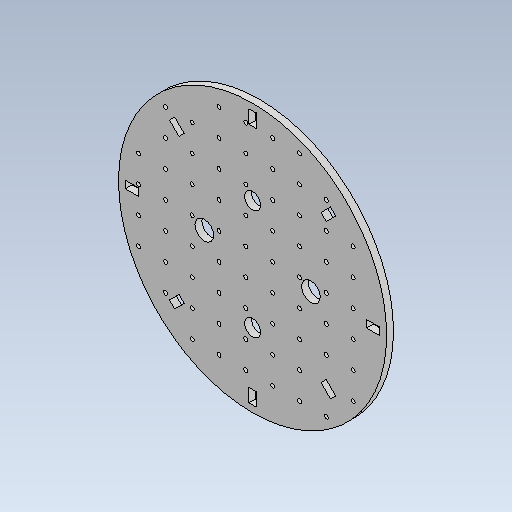
# Autodesk Inventor part: midPlate
Saved by Autodesk Inventor 2025 (Build 290162000, 162)
## iProperties
Created: 2024-08-12
Part Number: midPlate
Material: Polycarbonate, Clear
Document SubType Name: Modeling
Designer: PC
Density: 1.2 g/cm^3
Appearance: Default
Author: PC
Autodesk Inventor part; units mm, degrees
ref_plane "YZ Plane" through (0, 0, 0) normal (1, 0, 0) x (0, 1, 0)
ref_plane "XZ Plane" through (0, 0, 0) normal (0, 1, 0) x (-1, 0, 0)
ref_plane "XY Plane" through (0, 0, 0) normal (0, 0, 1) x (1, 0, 0)
sketch "Sketch1" plane through (0, 0, 0) normal (0, 0, 1) x (1, 0, 0)
  circle A0 centre (0, -18.52) radius 100
  line L0 (65, -83.52) -> (-65, -83.52) construction
  line L1 (-65, -83.52) -> (-65, 46.48) construction
  line L2 (-65, 46.48) -> (65, 46.48) construction
  line L3 (65, 46.48) -> (65, -83.52) construction
  line L4 (65, -83.52) -> (-65, 46.48) construction
  line L5 (-65, -83.52) -> (65, 46.48) construction
  line L6 (45, 26.48) -> (-45, 26.48) construction
  line L7 (-45, 26.48) -> (-45, -63.52) construction
  line L8 (-45, -63.52) -> (45, -63.52) construction
  line L9 (45, -63.52) -> (45, 26.48) construction
  line L10 (-25, 6.48) -> (25, 6.48) construction
  line L11 (25, 6.48) -> (25, -43.52) construction
  line L12 (25, -43.52) -> (-25, -43.52) construction
  line L13 (-25, -43.52) -> (-25, 6.48) construction
  line L14 (5, -13.52) -> (-5, -13.52) construction
  line L15 (-5, -13.52) -> (-5, -23.52) construction
  line L16 (-5, -23.52) -> (5, -23.52) construction
  line L17 (5, -23.52) -> (5, -13.52) construction
  circle A1 centre (-65, 46.48) radius 1.5
  circle A2 centre (-45, 46.48) radius 1.5
  circle A3 centre (-25, 46.48) radius 1.5
  circle A4 centre (-5, 46.48) radius 1.5
  circle A5 centre (15, 46.48) radius 1.5
  circle A6 centre (35, 46.48) radius 1.5
  circle A7 centre (55, 46.48) radius 1.5
  circle A8 centre (-65, 26.48) radius 1.5
  circle A9 centre (-65, 6.48) radius 1.5
  circle A10 centre (-65, -13.52) radius 1.5
  circle A11 centre (-65, -33.52) radius 1.5
  circle A12 centre (-65, -53.52) radius 1.5
  circle A13 centre (-65, -73.52) radius 1.5
  circle A14 centre (-45, 26.48) radius 1.5
  circle A15 centre (-25, 26.48) radius 1.5
  circle A16 centre (-5, 26.48) radius 1.5
  circle A17 centre (15, 26.48) radius 1.5
  circle A18 centre (35, 26.48) radius 1.5
  circle A19 centre (55, 26.48) radius 1.5
  circle A20 centre (-45, 6.48) radius 1.5
  circle A21 centre (-25, 6.48) radius 1.5
  circle A22 centre (-5, 6.48) radius 1.5
  circle A23 centre (15, 6.48) radius 1.5
  circle A24 centre (35, 6.48) radius 1.5
  circle A25 centre (55, 6.48) radius 1.5
  circle A26 centre (75, 6.48) radius 1.5
  circle A27 centre (-45, -13.52) radius 1.5
  circle A28 centre (-25, -13.52) radius 1.5
  circle A29 centre (-5, -13.52) radius 1.5
  circle A30 centre (15, -13.52) radius 1.5
  circle A31 centre (35, -13.52) radius 1.5
  circle A32 centre (55, -13.52) radius 1.5
  circle A33 centre (75, -13.52) radius 1.5
  circle A34 centre (-85, 6.48) radius 1.5
  circle A35 centre (-85, -13.52) radius 1.5
  circle A36 centre (-85, -33.52) radius 1.5
  circle A37 centre (-45, -33.52) radius 1.5
  circle A38 centre (-25, -33.52) radius 1.5
  circle A39 centre (-5, -33.52) radius 1.5
  circle A40 centre (15, -33.52) radius 1.5
  circle A41 centre (35, -33.52) radius 1.5
  circle A42 centre (55, -33.52) radius 1.5
  circle A43 centre (75, -33.52) radius 1.5
  circle A44 centre (-85, -53.52) radius 1.5
  circle A45 centre (-45, -53.52) radius 1.5
  circle A46 centre (-25, -53.52) radius 1.5
  circle A47 centre (-5, -53.52) radius 1.5
  circle A48 centre (15, -53.52) radius 1.5
  circle A49 centre (35, -53.52) radius 1.5
  circle A50 centre (55, -53.52) radius 1.5
  circle A51 centre (75, -53.52) radius 1.5
  circle A52 centre (-45, -73.52) radius 1.5
  circle A53 centre (-25, -73.52) radius 1.5
  circle A54 centre (-5, -73.52) radius 1.5
  circle A55 centre (15, -73.52) radius 1.5
  circle A56 centre (35, -73.52) radius 1.5
  circle A57 centre (55, -73.52) radius 1.5
  circle A58 centre (75, -73.52) radius 1.5
  circle A59 centre (75, 26.48) radius 1.5
  line L18 (0, -18.52) -> (0, 118.6528) construction
  line L19 (0, -18.52) -> (87, -18.52) construction
  circle A60 centre (0, 18.48) radius 6
  circle A61 centre (0, -63.52) radius 6
  circle A62 centre (-36, -18.52) radius 7
  circle A63 centre (43.5, -18.52) radius 7
  line L20 (-25, 46.48) -> (-25, 71.8994) construction
  circle A64 centre (-25, 66.48) radius 1.5
  circle A65 centre (-5, 66.48) radius 1.5
  circle A66 centre (15, 66.48) radius 1.5
  circle A67 centre (35, 66.48) radius 1.5
  circle A68 centre (-45, -93.52) radius 1.5
  circle A69 centre (-25, -93.52) radius 1.5
  circle A70 centre (-5, -93.52) radius 1.5
  circle A71 centre (15, -93.52) radius 1.5
  circle A72 centre (35, -93.52) radius 1.5
  circle A73 centre (55, -93.52) radius 1.5
  point P0 (0, 0)
  point P1 (-20, 81.3433)
  point P2 (-25.16, 81.3433)
  point P3 (-25, -18.52)
  dimension "d52" = 200
  dimension "d54" = 130
  dimension "d55" = 20
  dimension "d56" = 20
  dimension "d57" = 20
  dimension "d58" = 3
  dimension "d59" = 20
  dimension "d60" = 20
  dimension "d61" = 20
  dimension "d62" = 20
  dimension "d63" = 20
  dimension "d64" = 20
  dimension "d65" = 20
  dimension "d66" = 20
  dimension "d67" = 20
  dimension "d68" = 20
  dimension "d69" = 20
  dimension "d70" = 20
  dimension "d71" = 20
  dimension "d79" = 12
  dimension "d80" = 37
  dimension "d81" = 12
  dimension "d82" = 14
  dimension "d85" = 14
  dimension "d86" = 43.5
  dimension "d102" = 20
  dimension "d109" = 20
  dimension "d116" = 20
  dimension "d123" = 20
  dimension "d130" = 20
  dimension "d137" = 20
  dimension "d144" = 20
  dimension "d151" = 20
  dimension "d158" = 20
  dimension "d165" = 20
  constraints: 74 centre point, 42 end point, 14 horizontal, 13 vertical, 8 parallel, 5 midpoint, 4 perpendicular, 2 coincident, 1 point on line, 145 other
  measures "d52" diameter of A0
  measures "d54" distance of L1.start L1.end
  measures "d55" distance between parallel lines of L2 L6
  measures "d56" distance between parallel lines of L6 L10
  measures "d57" distance between parallel lines of L10 L14
  measures "d58" diameter of A1
  measures "d59" distance of A1.centre A2.centre
  measures "d60" distance of A1.centre A8.centre
  measures "d61" distance of A8.centre A14.centre
  measures "d62" distance of A9.centre A20.centre
  measures "d63" distance of A10.centre A27.centre
  measures "d64" distance of A9.centre A34.centre
  measures "d65" distance of A10.centre A35.centre
  measures "d66" distance of A11.centre A36.centre
  measures "d67" distance of A11.centre A37.centre
  measures "d68" distance of A12.centre A44.centre
  measures "d69" distance of A12.centre A45.centre
  measures "d70" distance of A13.centre A52.centre
  measures "d71" distance of A19.centre A59.centre
  measures "d79" diameter of A60
  measures "d80" distance of point (0, -18.52) A60.centre
  measures "d81" diameter of A61
  measures "d82" diameter of A62
  measures "d85" diameter of A63
  measures "d86" distance of point (0, -18.52) A63.centre
  measures "d102" distance of L20.start A64.centre
  measures "d109" distance of A4.centre A65.centre
  measures "d116" distance of A5.centre A66.centre
  measures "d123" distance of A6.centre A67.centre
  measures "d130" distance of A52.centre A68.centre
  measures "d137" distance of A53.centre A69.centre
  measures "d144" distance of A54.centre A70.centre
  measures "d151" distance of A55.centre A71.centre
  measures "d158" distance of A56.centre A72.centre
  measures "d165" distance of A57.centre A73.centre
extrude "Extrusion1" add sketch "Sketch1" along normal blind 5.1
sketch "Sketch2" plane through (0, -18.52, 5.1) normal (0, 0, 1) x (1, 0, 0)
  line L0 (-85, -2.75) -> (-95, -2.75)
  line L1 (-95, -2.75) -> (-95, 2.75)
  line L2 (-95, 2.75) -> (-85, 2.75)
  line L3 (-85, 2.75) -> (-85, -2.75)
  line L4 (-85, -2.75) -> (-95, 2.75) construction
  line L5 (-95, -2.75) -> (-85, 2.75) construction
  circle A0 centre (0, 0) radius 100 projected
  circle A1 centre (55, -75) radius 1.5 projected
  circle A2 centre (35, -75) radius 1.5 projected
  circle A3 centre (15, -75) radius 1.5 projected
  circle A4 centre (-5, -75) radius 1.5 projected
  circle A5 centre (-25, -75) radius 1.5 projected
  circle A6 centre (-45, -75) radius 1.5 projected
  circle A7 centre (35, 85) radius 1.5 projected
  circle A8 centre (15, 85) radius 1.5 projected
  circle A9 centre (-5, 85) radius 1.5 projected
  circle A10 centre (-25, 85) radius 1.5 projected
  circle A11 centre (-5, -35) radius 1.5 projected
  circle A12 centre (15, -35) radius 1.5 projected
  circle A13 centre (0, -45) radius 6 projected
  circle A14 centre (15, -55) radius 1.5 projected
  circle A15 centre (-5, -55) radius 1.5 projected
  circle A16 centre (75, -55) radius 1.5 projected
  circle A17 centre (75, -35) radius 1.5 projected
  circle A18 centre (55, -55) radius 1.5 projected
  circle A19 centre (35, -55) radius 1.5 projected
  circle A20 centre (55, -35) radius 1.5 projected
  circle A21 centre (35, -35) radius 1.5 projected
  circle A22 centre (75, -15) radius 1.5 projected
  circle A23 centre (55, -15) radius 1.5 projected
  circle A24 centre (35, -15) radius 1.5 projected
  circle A25 centre (15, -15) radius 1.5 projected
  circle A26 centre (-85, 25) radius 1.5 projected
  circle A27 centre (-45, 25) radius 1.5 projected
  circle A28 centre (-25, 25) radius 1.5 projected
  circle A29 centre (-85, 5) radius 1.5 projected
  circle A30 centre (-25, 5) radius 1.5 projected
  circle A31 centre (-45, 5) radius 1.5 projected
  circle A32 centre (-85, -15) radius 1.5 projected
  circle A33 centre (-65, -15) radius 1.5 projected
  circle A34 centre (-65, 5) radius 1.5 projected
  circle A35 centre (-65, 25) radius 1.5 projected
  circle A36 centre (-65, 45) radius 1.5 projected
  circle A37 centre (-65, 65) radius 1.5 projected
  circle A38 centre (-45, -15) radius 1.5 projected
  circle A39 centre (-36, 0) radius 7 projected
  circle A40 centre (-25, -15) radius 1.5 projected
  circle A41 centre (43.5, 0) radius 7 projected
  circle A42 centre (35, 5) radius 1.5 projected
  circle A43 centre (55, 5) radius 1.5 projected
  circle A44 centre (75, 5) radius 1.5 projected
  circle A45 centre (-25, -55) radius 1.5 projected
  circle A46 centre (-45, -55) radius 1.5 projected
  circle A47 centre (-65, -55) radius 1.5 projected
  circle A48 centre (-45, -35) radius 1.5 projected
  circle A49 centre (-25, -35) radius 1.5 projected
  circle A50 centre (-85, -35) radius 1.5 projected
  circle A51 centre (-65, -35) radius 1.5 projected
  circle A52 centre (75, 45) radius 1.5 projected
  circle A53 centre (75, 25) radius 1.5 projected
  circle A54 centre (55, 65) radius 1.5 projected
  circle A55 centre (55, 45) radius 1.5 projected
  circle A56 centre (35, 65) radius 1.5 projected
  circle A57 centre (15, 65) radius 1.5 projected
  circle A58 centre (35, 45) radius 1.5 projected
  circle A59 centre (55, 25) radius 1.5 projected
  circle A60 centre (15, 45) radius 1.5 projected
  circle A61 centre (35, 25) radius 1.5 projected
  circle A62 centre (0, 37) radius 6 projected
  circle A63 centre (-5, 5) radius 1.5 projected
  circle A64 centre (15, 5) radius 1.5 projected
  circle A65 centre (15, 25) radius 1.5 projected
  circle A66 centre (-5, -15) radius 1.5 projected
  circle A67 centre (-5, 25) radius 1.5 projected
  circle A68 centre (-45, 45) radius 1.5 projected
  circle A69 centre (-45, 65) radius 1.5 projected
  circle A70 centre (-25, 45) radius 1.5 projected
  circle A71 centre (-5, 45) radius 1.5 projected
  circle A72 centre (-25, 65) radius 1.5 projected
  circle A73 centre (-5, 65) radius 1.5 projected
  line L6 (-2.75, -95) -> (-2.75, -85)
  line L7 (-2.75, -85) -> (2.75, -85)
  line L8 (2.75, -85) -> (2.75, -95)
  line L9 (2.75, -95) -> (-2.75, -95)
  line L10 (95, -2.75) -> (85, -2.75)
  line L11 (85, -2.75) -> (85, 2.75)
  line L12 (85, 2.75) -> (95, 2.75)
  line L13 (95, 2.75) -> (95, -2.75)
  line L14 (2.75, 95) -> (2.75, 85)
  line L15 (2.75, 85) -> (-2.75, 85)
  line L16 (-2.75, 85) -> (-2.75, 95)
  line L17 (-2.75, 95) -> (2.75, 95)
  point P0 (0, 18.52)
  point P1 (-90, 0)
  point P2 (-95, 0)
  point P3 (-90, -2.75)
  point P4 (2.75, -90)
  point P5 (0, -95)
  point P6 (90, 2.75)
  point P7 (95, 0)
  point P8 (-2.75, 90)
  point P9 (0, 95)
  dimension "d176" = 90
  dimension "d177" = 95
  dimension "d178" = 2.75
  dimension "d181" = 360
  constraints: 36 end point, 4 midpoint, 2 parallel, 1 horizontal, 1 horizontal alignment, 1 perpendicular, 41 other
  measures "d176" distance of A0.centre point (-90, 0)
  measures "d177" distance of A0.centre point (-95, 0)
  measures "d178" vertical distance of A0.centre point (-90, -2.75)
extrude "Extrusion2" cut sketch "Sketch2" against normal blind 10 contours L0 L1 L2 L3 | L6 L7 L8 L9 | L10 L11 L12 L13 | L14 L15 L16 L17
sketch "Sketch3" plane through (0, -18.52, 5.1) normal (0, 0, 1) x (1, 0, 0)
  line L0 (0, 0) -> (-61.3465, 61.3465) construction
  line L1 (0, 0) -> (-16.1395, 0) construction
  line L2 (0, 0) -> (-21.5595, -21.5595) construction
  line L3 (-58.1261, 62.0152) -> (-51.055, 54.9441)
  line L4 (-62.0152, 58.1261) -> (-54.9441, 51.055)
  line L5 (-62.0152, 58.1261) -> (-58.1261, 62.0152)
  line L6 (-54.9441, 51.055) -> (-51.055, 54.9441)
  line L7 (0, 0) -> (61.3465, -61.3465) construction
  line L8 (62.0152, -58.1261) -> (54.9441, -51.055)
  line L9 (58.1261, -62.0152) -> (51.055, -54.9441)
  line L10 (58.1261, -62.0152) -> (62.0152, -58.1261)
  line L11 (51.055, -54.9441) -> (54.9441, -51.055)
  circle A0 centre (0, 0) radius 100 projected
  line L12 (54.9441, 51.055) -> (51.055, 54.9441)
  line L13 (62.0152, 58.1261) -> (54.9441, 51.055)
  line L14 (58.1261, 62.0152) -> (51.055, 54.9441)
  line L15 (0, 0) -> (61.3465, 61.3465) construction
  line L16 (62.0152, 58.1261) -> (58.1261, 62.0152)
  line L17 (-51.055, 54.9441) -> (-54.9441, 51.055)
  line L18 (-58.1261, 62.0152) -> (-51.055, 54.9441)
  line L19 (-62.0152, 58.1261) -> (-54.9441, 51.055)
  line L20 (0, 0) -> (-61.3465, 61.3465) construction
  line L21 (-58.1261, 62.0152) -> (-62.0152, 58.1261)
  line L22 (-54.9441, -51.055) -> (-51.055, -54.9441)
  line L23 (-62.0152, -58.1261) -> (-54.9441, -51.055)
  line L24 (-58.1261, -62.0152) -> (-51.055, -54.9441)
  line L25 (0, 0) -> (-61.3465, -61.3465) construction
  line L26 (-62.0152, -58.1261) -> (-58.1261, -62.0152)
  point P0 (0, 18.52)
  point P1 (-54.5906, 58.4797)
  point P2 (-58.4797, 54.5906)
  point P3 (58.4797, -54.5906)
  point P4 (54.5906, -58.4797)
  point P5 (54.5906, 58.4797)
  point P6 (58.4797, 54.5906)
  point P7 (-58.4797, 54.5906)
  point P8 (-54.5906, 58.4797)
  point P9 (-54.5906, -58.4797)
  point P10 (-58.4797, -54.5906)
  dimension "d185" = 45
  dimension "d186" = 45
  dimension "d187" = 10
  dimension "d191" = 18.5201
  dimension "d192" = 80
  dimension "d193" = 2.75
  dimension "d194" = 80
  dimension "d195" = 2.75
  dimension "d200" = 360
  constraints: 54 end point, 7 symmetric about line, 3 parallel, 2 midpoint, 1 horizontal, 1 vertical alignment, 53 other
  measures "d185" angle of L0 L1
  measures "d186" angle of L2 L1
  measures "d187" distance of L3.start L3.end
  measures "d191" distance of L0.start point (0, 18.52)
  measures "d192" distance of L0.start point (-54.591, 58.48)
  measures "d193" distance from line of L0 point (-54.591, 58.48)
  measures "d194" distance of L0.start point (-58.48, 54.591)
  measures "d195" distance from line of L0 point (-58.48, 54.591)
extrude "Extrusion3" cut sketch "Sketch3" against normal blind 10 contours L3 L6 L4 L5 | L10 L9 L11 L8
extrude "Extrusion4" cut sketch "Sketch3" against normal blind 10 contours L12 L14 L16 L13 | L22 L24 L26 L23
body "Solid1"
